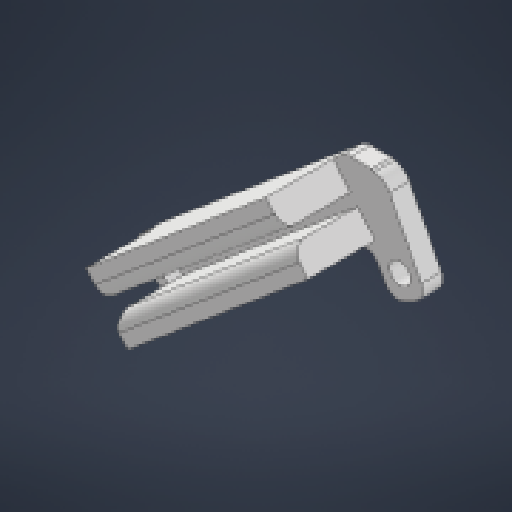
# Autodesk Inventor part: skr-mini-mount-clip
Saved by Autodesk Inventor 2025 (Build 290162000, 162)
## iProperties
Created: 2024-10-27
Part Number: skr-mini-mount-clip
Material: Generic
Document SubType Name: Modeling
Designer: Windows 7 was better
Density: 1 g/cm^3
Appearance: Default
Author: Windows 7 was better
Autodesk Inventor part; units mm, degrees
ref_plane "YZ Plane" through (0, 0, 0) normal (1, 0, 0) x (0, 1, 0)
ref_plane "XZ Plane" through (0, 0, 0) normal (0, 1, 0) x (-1, 0, 0)
ref_plane "XY Plane" through (0, 0, 0) normal (0, 0, 1) x (1, 0, 0)
sketch "Sketch1" plane through (0, 0, 0) normal (0, 0, 1) x (1, 0, 0)
  circle A0 centre (0.5705, 6.6467) radius 1.6 projected
  circle A1 centre (34.1954, 23.8887) radius 1.6 projected
  circle A2 centre (-47.845, -32.335) radius 1.55 projected
  circle A3 centre (-32.175, 32.335) radius 1.55 projected
  circle A4 centre (16.035, -5.485) radius 1.55 projected
  circle A5 centre (29.985, 32.135) radius 1.55 projected
  circle A6 centre (47.845, -2.845) radius 1.55 projected
  line L0 (41.7829, 2.4307) -> (31.0323, 23.4866) projected
  line L1 (17.7425, -2.333) -> (40.1671, -0.4719) projected
  line L2 (1.7387, 9.5432) -> (3.1056, 8.4709) projected
  line L3 (8.2098, 7.5322) -> (27.9655, 24.1092) projected
  line L4 (27.8513, 29.235) -> (3.1056, 8.4709) projected
  line L5 (1.7387, 9.5432) -> (25.2065, 29.235) projected
  line L6 (27.8513, 29.235) -> (25.2065, 29.235) projected
  line L7 (14.7743, 25.7029) -> (-0.2342, 13.1093) projected
  line L8 (-18.8076, 25.6614) -> (-2.7542, 13.0678) projected
  line L9 (13.4887, 29.235) -> (-17.5731, 29.235) projected
  line L10 (7.493, -2.5969) -> (-27.9115, 25.1774) projected
  line L11 (-39.8787, -25.7324) -> (7.0335, -6.0143) projected
  line L12 (-31.0897, 24.0748) -> (-42.5975, -23.4177) projected
  line L13 (16.4652, -8.5584) -> (-46.6826, -35.1006) projected
  line L14 (48.0931, -5.8347) -> (17.0747, -8.409) projected
  arc A7 (48.0931, -5.8347) -> (50.5169, -1.4808) centre (47.845, -2.845) ccw projected
  line L15 (32.6569, 33.4992) -> (50.5169, -1.4808) projected
  arc A8 (32.6569, 33.4992) -> (29.985, 35.135) centre (29.985, 32.135) ccw projected
  line L16 (29.985, 35.235) -> (29.985, 35.135) projected
  line L17 (-31.4069, 35.235) -> (29.985, 35.235) projected
  arc A9 (-31.4069, 35.235) -> (-35.0906, 33.0415) centre (-32.175, 32.335) ccw projected
  line L18 (-50.7606, -31.6285) -> (-35.0906, 33.0415) projected
  arc A10 (-50.7606, -31.6285) -> (-46.6826, -35.1006) centre (-47.845, -32.335) ccw projected
  line L19 (29.8899, 25.724) -> (34.6062, 29.6814)
  line L20 (18.9837, 29.235) -> (26.1342, 35.235)
  line L21 (-1.4774, 12.0662) -> (-6.1744, 8.1249)
  line L22 (6.3217, 5.9479) -> (1.6247, 2.0067)
  line L23 (34.1954, 23.8887) -> (35.4353, 20.9387)
  line L24 (35.4353, 20.9387) -> (32.9746, 19.6824)
  line L25 (35.4353, 20.9387) -> (38.3184, 22.4108)
  arc A11 (16.3427, -1.9134) -> (17.7425, -2.333) centre (17.5771, -0.3398) ccw projected
  line L26 (8.261, 4.4266) -> (16.3427, -1.9134) projected
  arc A12 (8.2098, 7.5322) -> (8.261, 4.4266) centre (9.4954, 6.0002) ccw projected
  arc A13 (31.0323, 23.4866) -> (27.9655, 24.1092) centre (29.251, 22.5771) ccw projected
  arc A14 (40.1671, -0.4719) -> (41.7829, 2.4307) centre (40.0017, 1.5213) ccw projected
  arc A15 (-2.7542, 13.0678) -> (-0.2342, 13.1093) centre (-1.5198, 14.6414) ccw projected
  arc A16 (-17.5731, 29.235) -> (-18.8076, 25.6614) centre (-17.5731, 27.235) ccw projected
  arc A17 (14.7743, 25.7029) -> (13.4887, 29.235) centre (13.4887, 27.235) ccw projected
  arc A18 (7.0335, -6.0143) -> (7.493, -2.5969) centre (6.2586, -4.1705) ccw projected
  arc A19 (-42.5975, -23.4177) -> (-39.8787, -25.7324) centre (-40.6537, -23.8886) ccw projected
  arc A20 (-27.9115, 25.1774) -> (-31.0897, 24.0748) centre (-29.1459, 23.6038) ccw projected
  arc A21 (17.0747, -8.409) -> (16.4652, -8.5584) centre (17.2401, -10.4022) ccw projected
  line L27 (18.9837, 29.235) -> (-1.4774, 12.0662)
  line L28 (6.2586, 5.8949) -> (29.8899, 25.724)
  point P0 (0, 0)
  dimension "d11" = 3.2
  constraints: 18 end point, 11 point on line, 1 parallel, 1 perpendicular
  measures "d11" distance of L23.start L23.end
extrude "Extrusion1" add sketch "Sketch1" along normal blind 3 contours A5 | L0 A13 L28 L19 L15 L25 L24 | L3 L28 L22 L10 L21 L27 L7 L20 L17 L16 A8 L15 L19 | L5 L6 L4 L2
fillet "Fillet1" radius 2 3 edges at (26.1342, 35.235, 1.5) (1.6247, 2.0067, 1.5) (-6.1744, 8.1249, 1.5)
sketch "Sketch2" plane through (0, 0, 3) normal (0, 0, 1) x (1, 0, 0)
  line L0 (1.7387, 9.5432) -> (25.2065, 29.235) construction
  line L1 (13.4726, 19.3891) -> (14.5654, 18.0868) construction
  line L2 (27.8513, 29.235) -> (3.1056, 8.4709) construction
  line L3 (1.1596, 6.838) -> (27.9712, 29.3356) construction
  line L4 (27.9712, 29.3356) -> (26.8784, 30.6379) construction
  line L5 (26.8784, 30.6379) -> (0.0669, 8.1403) construction
  line L6 (0.0669, 8.1403) -> (1.1596, 6.838) construction
  line L7 (1.1596, 6.838) -> (26.8784, 30.6379) construction
  line L8 (27.9712, 29.3356) -> (0.0669, 8.1403) construction
  line L9 (1.1596, 6.838) -> (36.1596, 6.838) construction
  line L10 (1.1596, 6.838) -> (27.9712, 29.3356)
  line L11 (27.9712, 29.3356) -> (30.5423, 26.2714)
  line L12 (30.5423, 26.2714) -> (3.7308, 3.7738)
  line L13 (3.7308, 3.7738) -> (1.1596, 6.838)
  line L14 (0.0669, 8.1403) -> (26.8784, 30.6379)
  line L15 (26.8784, 30.6379) -> (24.3073, 33.702)
  line L16 (24.3073, 33.702) -> (-2.5043, 11.2045)
  line L17 (-2.5043, 11.2045) -> (0.0669, 8.1403)
  circle A0 centre (0.5705, 6.6467) radius 1.6 projected
  point P0 (0, 0)
  point P1 (14.019, 18.7379)
  point P2 (0.0505, 8.1598)
  point P3 (0.1146, 8.1803)
  point P4 (1.9324, 7.4865)
  point P5 (1.9704, 5.8718)
  dimension "d3" = 35
  dimension "d4" = 40
  dimension "d5" = 1.7
  dimension "d6" = 4
  dimension "d7" = 4
  constraints: 32 end point, 6 parallel, 4 midpoint, 3 collinear, 3 perpendicular, 1 equal length, 1 horizontal, 1 point on line
  measures "d3" distance of L3.start L3.end
  measures "d4" angle of L9 L3
  measures "d5" distance of L4.end L3.end
  measures "d6" distance of L3.end L11.end
  measures "d7" distance of L15.end L4.end
extrude "Extrusion2" add sketch "Sketch2" along normal blind 10 contours L10 L11 L12 L13 A0 | A0 L17 L16 L15 L14
fillet "Fillet2" radius 2 2 edges at (14.9518, 18.411, 13) (13.4965, 19.4091, 13)
fillet "Fillet3" radius 2 2 edges at (38.3184, 22.4108, 1.5) (32.9746, 19.6824, 1.5)
fillet "Fillet4" radius 2 1 edges at (29.985, 35.135, 1.5)
body "Solid1"
